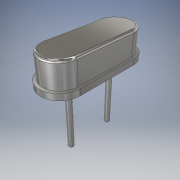
# Autodesk Inventor part: Crystal
Saved by Autodesk Inventor 2018 (Build 220112000, 112)
## iProperties
Created: 2021-02-07
Part Number: Crystal
Material: Všeobecné
Document SubType Name: Modeling
Designer: Jozko Mrkvicka
Density: 1 g/cm^3
Appearance: Výchozí
Author: Jozko Mrkvicka
Autodesk Inventor part; units mm, degrees
ref_plane "YZ Plane" through (0, 0, 0) normal (1, 0, 0) x (0, 1, 0)
ref_plane "XZ Plane" through (0, 0, 0) normal (0, 1, 0) x (-1, 0, 0)
ref_plane "XY Plane" through (0, 0, 0) normal (0, 0, 1) x (1, 0, 0)
sketch "Náčrt1" plane through (0, 0, 0) normal (0, 1, 0) x (-1, 0, 0)
  line L0 (4.445, -2.2225) -> (4.445, -8.5725)
  line L1 (0, -8.5725) -> (0, -2.2225)
  arc A0 (0, -8.5725) -> (4.445, -8.5725) centre (2.2225, -8.5725) ccw
  arc A1 (4.445, -2.2225) -> (0, -2.2225) centre (2.2225, -2.2225) ccw
  point P0 (0, 0)
  dimension "d2" = 4.445
  dimension "d3" = 4.445
  constraints: 4 end point, 4 point on circle, 2 centre point, 1 parallel, 2 other
  measures "d2" diameter of A1
  measures "d3" diameter of A0
extrude "Vysunutí1" add sketch "Náčrt1" along normal blind 0.635
sketch "Náčrt2" plane through (0, 0.635, 0) normal (0, 1, 0) x (1, 0, 0)
  arc A0 (0, 8.5725) -> (-4.445, 8.5725) centre (-2.2225, 8.5725) ccw projected
  arc A1 (-4.445, 2.2225) -> (0, 2.2225) centre (-2.2225, 2.2225) ccw projected
  arc A2 (-4.1275, 2.2225) -> (-0.3175, 2.2225) centre (-2.2225, 2.2225) ccw
  arc A3 (-0.3175, 8.5725) -> (-4.1275, 8.5725) centre (-2.2225, 8.5725) ccw
  line L0 (-4.1275, 2.2225) -> (-4.1275, 8.5725)
  line L1 (-0.3175, 8.5725) -> (-0.3175, 2.2225)
  point P0 (0, 0)
  point P1 (-2.2225, 5.3975)
  constraints: 4 end point, 4 point on circle, 2 centre point, 2 coincident, 1 parallel
extrude "Vysunutí2" add sketch "Náčrt2" along normal blind 2.54
fillet "Zaoblení1" radius 0.254 4 edges at (-2.2225, 3.175, -10.4775) (-4.1275, 3.175, -5.3975) (-2.2225, 3.175, -0.3175) (-0.3175, 3.175, -5.3975)
sketch "Náčrt3" plane through (0, 0, 0) normal (0, -1, 0) x (1, 0, 0)
  circle A0 centre (-2.2225, -2.8575) radius 0.9525
  circle A1 centre (-2.2225, -7.9375) radius 0.9525
  point P0 (0, 0)
  dimension "d12" = 1.905
  dimension "d13" = 1.905
  constraints: 2 centre point
  measures "d12" diameter of A0
  measures "d13" diameter of A1
extrude "Vysunutí3" cut sketch "Náčrt3" against normal blind 0.0635
sketch "Náčrt4" plane through (-2.2225, 0.0635, -2.8575) normal (0, -1, 0) x (1, 0, 0)
  circle A0 centre (0, 0) radius 0.9525 projected
  circle A1 centre (0, 0) radius 0.3175
  circle A2 centre (0, -5.08) radius 0.9525 projected
  circle A3 centre (0, -5.08) radius 0.3175
  point P0 (2.2225, 2.8575)
  dimension "d16" = 0.635
  constraints: 2 centre point, 2 coincident
  measures "d16" diameter of A1
extrude "Vysunutí4" add sketch "Náčrt4" along normal blind 7.62 contours A1 | A3
fillet "Zaoblení2" radius 0.254 2 edges at (-2.54, -7.5565, -2.8575) (-2.54, -7.5565, -7.9375)
